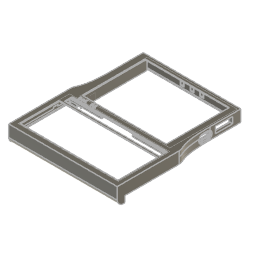
sol.01 (Autodesk Fusion 360 design; units mm, degrees)
Autodesk Fusion 360 part; units mm, degrees
note: some values were not read from the file. Set by a fixed rule: which face or edge a step refers to.
(part 1 of 2)
sketch "Sketch1" plane through (0, 0, 0) normal (0, 0, 1) x (1, 0, 0)
  line L0 (11.705, 132.02) -> (105.005, 132.02)
  line L1 (105.005, 132.02) -> (105.005, 61.35)
  line L2 (105.005, 61.35) -> (11.705, 61.35)
  line L3 (11.705, 61.35) -> (11.705, 132.02)
  line L4 (4.4, 58.89) -> (108.3, 58.89)
  line L5 (108.3, 58.89) -> (108.3, 5.46)
  line L6 (108.3, 5.46) -> (4.4, 5.46)
  line L7 (4.4, 5.46) -> (4.4, 58.89)
  line L8 (2, 62.35) -> (110.7, 62.35)
  line L9 (110.7, 62.35) -> (110.7, 2)
  line L10 (110.7, 2) -> (2, 2)
  line L11 (2, 2) -> (2, 62.35)
  line L12 (12.895, 129.09) -> (99.805, 129.09)
  line L13 (99.805, 129.09) -> (99.805, 63.79)
  line L14 (99.805, 63.79) -> (12.895, 63.79)
  line L15 (12.895, 63.79) -> (12.895, 129.09)
  line L16 (12.895, 129.09) -> (99.805, 63.79) construction
  line L17 (4.4, 58.89) -> (108.3, 5.46) construction
  line L18 (2, 62.35) -> (110.7, 2) construction
  line L19 (56.35, 96.44) -> (56.35, 32.175) construction
  line L20 (0, 0) -> (112.7, 0)
  line L21 (5.695, 64.35) -> (107.005, 64.35) construction
  line L22 (107.005, 134.02) -> (107.005, 70.045)
  line L23 (5.695, 134.02) -> (5.695, 70.045)
  line L24 (112.7, 0) -> (112.7, 64.35)
  line L25 (0, 64.35) -> (0, 0)
  line L26 (107.005, 134.02) -> (5.695, 134.02)
  line L27 (0, 64.35) -> (5.695, 70.045)
  line L28 (5.695, 64.35) -> (7.3315, 64.35) construction
  line L29 (112.7, 64.35) -> (107.005, 70.045)
  line L30 (107.005, 64.35) -> (105.9795, 64.35) construction
  line L31 (112.7, 64.35) -> (107.005, 64.35) construction
  line L32 (107.005, 64.35) -> (112.7, 64.35) construction
  line L33 (0, 64.35) -> (5.695, 64.35) construction
  line L34 (5.695, 70.045) -> (5.695, 64.35) construction
  line L35 (107.005, 70.045) -> (107.005, 64.35) construction
  line L36 (0, 64.35) -> (5.695, 64.35) construction
  line L37 (107.25, 47.24) -> (5.45, 47.24)
  line L38 (5.45, 47.24) -> (5.45, 6.29)
  line L39 (5.45, 6.29) -> (107.25, 6.29)
  line L40 (107.25, 6.29) -> (107.25, 47.24)
  line L41 (107.25, 57.36) -> (8.65, 57.36)
  line L42 (8.65, 57.36) -> (8.65, 49.36)
  line L43 (8.65, 49.36) -> (107.25, 49.36)
  line L44 (107.25, 49.36) -> (107.25, 57.36)
  line L45 (0, 64.35) -> (0, 70.045) construction
  line L46 (0, 70.045) -> (5.695, 70.045) construction
  line L47 (5.695, 70.045) -> (5.695, 102.0325) construction
  spline S0 degree 3 poles (0, 64.35) (0, 70.045) (5.695, 70.045) (5.695, 102.0325) knots 0 0 0 0 1 1 1 1
  line L48 (112.7, 64.35) -> (112.7, 70.045) construction
  line L49 (112.7, 70.045) -> (107.005, 70.045) construction
  line L50 (107.005, 70.045) -> (107.005, 102.0325) construction
  spline S1 degree 3 poles (112.7, 64.35) (112.7, 70.045) (107.005, 70.045) (107.005, 102.0325) knots 0 0 0 0 1 1 1 1
  point P0 (56.35, 96.44)
  point P1 (56.35, 32.175)
  point P2 (56.35, 32.175)
  dimension "d1" = 93.3
  dimension "d2" = 70.67
  dimension "d3" = 103.9
  dimension "d4" = 53.43
  dimension "d5" = 108.7
  dimension "d6" = 60.35
  dimension "d7" = 86.91
  dimension "d8" = 65.3
  dimension "d9" = 67.74
  dimension "d10" = 88.1
  dimension "d11" = 1
  dimension "d12" = 2
  dimension "d14" = 2
  dimension "d17" = 2
  dimension "d19" = 45
  dimension "d20" = 45
  dimension "d21" = 2
  dimension "d22" = 2
  dimension "d45" = 40.95
  dimension "d46" = 101.8
  dimension "d47" = 0.83
  dimension "d48" = 1.05
  dimension "d49" = 8
  dimension "d50" = 98.6
  dimension "d52" = 1.53
  dimension "d54" = 1.05
  dimension "d55" = 2
  constraint horizontal L0
  constraint vertical L1
  constraint horizontal L2
  constraint vertical L3
  constraint horizontal L4
  constraint vertical L5
  constraint horizontal L6
  constraint vertical L7
  constraint horizontal L8
  constraint vertical L9
  constraint horizontal L10
  constraint vertical L11
  constraint horizontal L12
  constraint vertical L13
  constraint horizontal L14
  constraint vertical L15
  constraint midpoint L16 P0
  constraint midpoint L17 P2
  constraint midpoint L18 P2
  constraint coincident P0 L19.start
  constraint coincident P2 P1
  constraint coincident P2 L19
  constraint vertical L19
  constraint horizontal L20
  constraint vertical L24
  constraint perpendicular L21 L24
  constraint perpendicular L21 L22
  constraint perpendicular L21 L23
  constraint vertical L25
  constraint horizontal L28
  constraint horizontal L30
  constraint perpendicular L24 L32
  constraint perpendicular L21 L34
  constraint perpendicular L21 L35
  constraint perpendicular L24 L36
  constraint equal L31 L36
  constraint coincident L20.start L25.end
  constraint horizontal L37
  constraint vertical L38
  constraint horizontal L39
  constraint vertical L40
  constraint horizontal L41
  constraint vertical L42
  constraint horizontal L43
  constraint vertical L44
  constraint vertical L45
  constraint coincident L23.end L27.end
  constraint horizontal L46
  constraint midpoint L23 L47.end
  constraint vertical L48
  constraint coincident L22.end L29.end
  constraint horizontal L49
  constraint midpoint L22 L50.end
  measures "d1" distance of L0.start L0.end
  measures "d2" distance of L0.start L2.end
  measures "d3" distance of L4.start L4.end
  measures "d4" distance of L4.start L6.end
  measures "d5" distance of L8.start L8.end
  measures "d6" distance of L8.start L10.end
  measures "d7" distance of L12.start L12.end
  measures "d8" distance of L12.start L14.end
  measures "d9" distance of L2 L12
  measures "d10" distance of L3 L13
  measures "d11" distance of L2 L8
  measures "d12" distance of L9 L24
  measures "d14" distance of L10 L20
  measures "d17" distance of L8 L21
  measures "d19" angle of L27 L28
  measures "d20" angle of L29 L30
  measures "d21" distance of L11 L25
  measures "d22" distance of L0 L26
  measures "d45" distance of L37.start L39.end
  measures "d46" distance of L37.start L37.end
  measures "d47" distance of L6 L39
  measures "d48" distance of L5 L40
  measures "d49" distance of L41.end L42.end
  measures "d50" distance of L41.start L41.end
  measures "d52" distance of L4 L41
  measures "d54" distance of L5 L44
  measures "d55" distance of L1 L22
sketch "Sketch2" plane through (0, 0, 0) normal (1, 0, 0) x (0, 1, 0)
  line L0 (64.35, 0) -> (70.045, 0)
  line L1 (64.35, 0) -> (0, 0)
  line L2 (0, 0) -> (64.35, 0)
  line L3 (64.35, 0) -> (70.045, 0)
  line L4 (134.02, 0) -> (70.045, 0)
  line L5 (134.02, 0) -> (70.045, 0)
  line L6 (0, 0) -> (134.52, 0)
  line L7 (134.52, 0) -> (134.52, 12.2)
  line L8 (134.52, 12.2) -> (0, 12.2)
  line L9 (0, 12.2) -> (0, 0)
  line L10 (129.09, 0) -> (63.79, 0)
  line L11 (63.79, 0) -> (129.09, 0)
  line L12 (129.55, 12.2) -> (66.3267, 12.2)
  line L13 (129.55, 12.2) -> (64.25, 12.2)
  line L14 (64.25, 12.2) -> (64.25, 11.45)
  line L15 (64.25, 11.45) -> (129.55, 11.45)
  line L16 (129.55, 11.45) -> (129.55, 12.2)
  line L17 (132.02, 0) -> (62.35, 0)
  line L18 (62.35, 0) -> (62.35, 11.45)
  line L19 (62.35, 11.45) -> (132.02, 11.45)
  line L20 (132.02, 11.45) -> (132.02, 0)
  line L21 (5.46, 0) -> (58.89, 0)
  line L22 (58.89, 0) -> (5.46, 0)
  line L23 (58.89, 0) -> (62.35, 0)
  line L24 (62.35, 0) -> (62.35, 6.9)
  line L25 (62.35, 6.9) -> (58.89, 6.9)
  line L26 (58.89, 6.9) -> (58.89, 0)
  line L27 (62.35, 0) -> (2, 0)
  line L28 (2, 0) -> (62.35, 0)
  line L29 (2, 0) -> (6.61, 0)
  line L30 (6.61, 0) -> (6.61, 6.9)
  line L31 (6.61, 6.9) -> (2, 6.9)
  line L32 (2, 6.9) -> (2, 0)
  line L33 (58.89, 0) -> (6.61, 0)
  line L34 (6.61, 0) -> (6.61, 12.2)
  line L35 (6.61, 12.2) -> (58.89, 12.2)
  line L36 (58.89, 12.2) -> (58.89, 0)
  point P0 (134.02, 0)
  point P1 (61.35, 0)
  point P2 (132.02, 0)
  point P3 (63.79, 0)
  point P4 (129.09, 0)
  point P5 (5.46, 0)
  point P6 (58.89, 0)
  point P7 (62.35, 0)
  point P8 (2, 0)
  dimension "d27" = 0.75
  dimension "d28" = 5.3
  dimension "d29" = 5.3
  dimension "d213" = 12.2
  constraint horizontal L6
  constraint vertical L7
  constraint horizontal L8
  constraint vertical L9
  constraint coincident L1.end L2.start
  constraint coincident L8 L12.start
  constraint coincident L8 L12.end
  constraint horizontal L13
  constraint vertical L14
  constraint horizontal L15
  constraint vertical L16
  constraint horizontal L17
  constraint vertical L18
  constraint horizontal L19
  constraint vertical L20
  constraint coincident P2 L17.start
  constraint coincident L14.end L19
  constraint horizontal L23
  constraint vertical L24
  constraint horizontal L25
  constraint vertical L26
  constraint coincident L18 L24.end
  constraint coincident P6 L21.end
  constraint horizontal L29
  constraint vertical L30
  constraint horizontal L31
  constraint vertical L32
  constraint coincident P8 L27.end
  constraint horizontal L33
  constraint vertical L34
  constraint horizontal L35
  constraint vertical L36
  constraint coincident L8 L34.end
  measures "d27" distance of L12.start L15.end
  measures "d28" distance of L8 L25
  measures "d29" distance of L8 L31
  measures "d213" distance of L1.end L8.end
extrude "Extrude1" add sketch "Sketch1" along normal up to surface (6.9 mm away) contours L20 L22 L23 L24 L25 L26 L27 L29 | L23 L27 S0 | L22 L29 S1 makes body 1
extrude "Extrude2" add sketch "Sketch1" along normal up to surface (4.55 mm away) from surface at 6.9 contours L1 L2 L3 L8 | L1 L2 L3 L8 L9 L10 L11 | L20 L22 L23 L24 L25 L26 L27 L29 | L23 L27 S0 | L22 L29 S1 bodies 1
extrude "Extrude3" add sketch "Sketch1" along normal up to surface (0.75 mm away) from surface at 11.45 contours L0 L1 L3 L8 | L1 L2 L3 L8 | L1 L2 L3 L8 L9 L10 L11 | L4 L5 L6 L7 | L20 L22 L23 L24 L25 L26 L27 L29 | L23 L27 S0 | L22 L29 S1 bodies 1
chamfer "Chamfer1" distance 15.9974 distance2 5.557 1 edges at (105.005, 62.35, 3.45) measured on face at (105.005, 108.7967, 6.1167) tangent chain off on bodies 1
sketch "Sketch4" plane through (0, 0, 6.9) normal (0, 0, -1) x (1, 0, 0)
  line L0 (2, -62.35) -> (11.705, -62.35)
  line L1 (11.705, -62.35) -> (105.005, -62.35)
  line L2 (105.005, -62.35) -> (105.005, -78.3474)
  line L3 (105.005, -78.3474) -> (110.562, -62.35)
  line L4 (110.562, -62.35) -> (110.7, -62.35)
  line L5 (110.7, -62.35) -> (110.7, -2)
  line L6 (110.7, -2) -> (2, -2)
  line L7 (2, -2) -> (2, -62.35)
  line L8 (108.3, -5.46) -> (108.3, -58.89)
  line L9 (108.3, -58.89) -> (4.4, -58.89)
  line L10 (4.4, -58.89) -> (4.4, -5.46)
  line L11 (4.4, -5.46) -> (108.3, -5.46)
  line L12 (108.3, -45.623) -> (114.9584, -45.623) construction
  line L13 (108.3, -43.4637) -> (114.9584, -43.4637) construction
  line L14 (4.4, -5.46) -> (108.3, -5.46)
  line L15 (4.4211, -57.9322) -> (38.5072, -57.9322)
  line L16 (4.4211, -5.46) -> (4.4211, -18.9792)
  line L17 (18.0884, -18.9792) -> (4.4211, -18.9792)
  line L18 (18.0884, -18.9792) -> (18.0884, -23.4975)
  line L19 (18.0884, -23.4975) -> (46.0418, -23.4975)
  line L20 (46.0418, -23.4975) -> (46.0418, -35.9296)
  line L21 (46.0418, -35.9296) -> (55.7614, -35.9296)
  line L22 (55.7614, -35.9296) -> (55.7614, -27.3401)
  line L23 (55.7614, -27.3401) -> (96.5989, -27.3401)
  line L24 (96.5989, -27.3401) -> (96.5989, -37.5118)
  line L25 (96.5989, -37.5118) -> (70.3785, -37.5118)
  line L26 (70.3785, -37.5118) -> (70.3785, -62.35)
  line L27 (38.5072, -62.35) -> (70.3785, -62.35)
  line L28 (70.3785, -62.35) -> (70.3785, -56.725)
  line L29 (38.5072, -56.725) -> (38.5072, -62.35)
  line L30 (70.3785, -56.725) -> (38.5072, -56.725)
  line L31 (4.0998, -44.4778) -> (-1.4115, -38.9664)
  line L32 (4.0998, -44.4778) -> (4.0998, -44.999)
  line L33 (-1.4116, -50.5103) -> (-1.4115, -38.9664)
  line L34 (4.0998, -44.999) -> (-1.4116, -50.5103)
  line L35 (2, -47.0988) -> (4.4, -47.0988)
  line L36 (2, -42.378) -> (4.4, -42.3611)
  line L37 (4.4211, -18.9792) -> (4.4211, -57.9322)
  line L38 (4.4, -47.0988) -> (4.4211, -47.0988)
  line L39 (4.4, -42.3611) -> (4.4211, -42.3611)
  line L40 (70.3785, -57.9438) -> (108.3, -57.9438)
  line L41 (108.3, -5.46) -> (108.3, -57.9438)
  line L42 (108.2, -57.9438) -> (108.2, -5.46)
  line L43 (108.3, -5.56) -> (4.4211, -5.56)
  dimension "d90" = 0.1
  dimension "d91" = 0.1
  constraint horizontal L12
  constraint coincident L8 L12.start
  constraint horizontal L13
  constraint coincident L8 L13.start
  constraint coincident L10.end L11.start
  constraint coincident L8.start L11.end
  constraint coincident L15.end L29
  constraint perpendicular L15 L29
  constraint parallel L26 L28
  constraint coincident L34 L35.start
  constraint coincident L7 L35.start
  constraint coincident L10 L35.end
  constraint coincident L31 L36.start
  constraint coincident L7 L36.start
  constraint coincident L10 L36.end
  constraint coincident L14 L16.start
  constraint vertical L16
  constraint horizontal L17
  constraint vertical L18
  constraint horizontal L19
  constraint vertical L20
  constraint horizontal L21
  constraint vertical L22
  constraint horizontal L23
  constraint vertical L24
  constraint horizontal L25
  constraint vertical L26
  constraint horizontal L30
  constraint vertical L29
  constraint vertical L37
  constraint coincident L37 L38.end
  constraint perpendicular L37 L38
  constraint coincident L37 L39.end
  constraint perpendicular L37 L39
  constraint coincident L26 L40.start
  constraint coincident L8 L40.end
  constraint perpendicular L8 L40
  constraint coincident L40 L42.start
  constraint coincident L14 L42.end
  constraint perpendicular L14 L42
  constraint coincident L41 L43.start
  constraint coincident L16 L43.end
  constraint perpendicular L16 L43
  measures "d90" distance of L14 L43
  measures "d91" distance of L41 L42
box "BoxPrimitive6" add length 1.8 width 103.9 height 1 placed x (0, 0, 1) y (-1, 0, 0) z (0, -1, 0) at (108.3, 58.89, 6.9) bodies 1
extrude "Extrude4" cut sketch "Sketch4" against normal blind 1.8 contours L1 L9 L26 L27 L28 L29 | L9 L26 L28 L29 L30 bodies 1
extrude "Extrude5" cut sketch "Sketch4" along normal blind 0.9639 and the other way blind 1.628 contours L7 L31 L33 L34 | L7 L31 L32 L34 | L10 L31 L32 L34 L35 L36 bodies 1
extrude "Extrude6" add sketch "Sketch4" against normal blind 1 separate body contours L16 L17 L18 L19 L20 L21 L22 L23 L24 L25 L26 L28 L40 L42 L43 makes body 2
sketch "Sketch6" plane through (0, 0, 11.45) normal (0, 0, -1) x (1, 0, 0)
  line L0 (99.805, -63.79) -> (99.805, -129.09)
  line L1 (99.805, -129.09) -> (12.895, -129.09)
  line L2 (12.895, -129.09) -> (12.895, -63.79)
  line L3 (12.895, -63.79) -> (99.805, -63.79)
  line L4 (105.005, -62.35) -> (11.705, -62.35)
  line L5 (11.705, -62.35) -> (11.705, -132.02)
  line L6 (11.705, -132.02) -> (105.005, -132.02)
  line L7 (105.005, -132.02) -> (105.005, -62.35)
  line L8 (105.005, -102.5509) -> (110.748, -108.2939)
  line L9 (105.005, -102.5509) -> (113.1461, -102.5509) construction
  line L10 (105.005, -91.9597) -> (113.3226, -83.6421)
  line L11 (105.005, -102.5509) -> (105.005, -91.9597)
  line L12 (110.748, -108.2939) -> (110.748, -86.2167)
  line L13 (105.005, -123.4211) -> (110.0091, -128.4252)
  line L14 (105.005, -123.4211) -> (112.0734, -123.4211) construction
  line L15 (105.005, -123.4211) -> (105.005, -109.5726)
  line L16 (70.1416, -132.02) -> (66.6021, -132.02)
  line L17 (66.6021, -132.02) -> (66.6021, -134.703)
  line L18 (66.6021, -134.703) -> (70.1416, -134.703)
  line L19 (70.1416, -134.703) -> (70.1416, -132.02)
  line L20 (60.0287, -132.02) -> (56.5904, -132.02)
  line L21 (56.5904, -132.02) -> (56.5904, -135.0064)
  line L22 (56.5904, -135.0064) -> (60.0287, -135.0064)
  line L23 (60.0287, -135.0064) -> (60.0287, -132.02)
  line L24 (49.8148, -132.02) -> (46.2753, -132.02)
  line L25 (46.2753, -132.02) -> (46.2753, -134.6019)
  line L26 (46.2753, -134.6019) -> (49.8148, -134.6019)
  line L27 (49.8148, -134.6019) -> (49.8148, -132.02)
  line L28 (11.705, -62.35) -> (10.905, -62.35)
  line L29 (10.905, -62.35) -> (10.905, -78.35)
  line L30 (10.905, -78.35) -> (6.705, -78.35)
  line L31 (6.705, -78.35) -> (6.705, -72.35)
  line L32 (6.705, -72.35) -> (8.405, -72.35)
  line L33 (8.405, -72.35) -> (8.405, -62.35)
  line L34 (8.405, -62.35) -> (11.705, -62.35)
  line L35 (8.405, -62.35) -> (10.905, -62.35)
  line L36 (6.705, -75.35) -> (5.2663, -75.35)
  line L37 (11.705, -63.3036) -> (10.905, -63.3036)
  line L38 (105.005, -109.5726) -> (107.7995, -106.7781)
  line L39 (107.7995, -106.7781) -> (107.7995, -126.2156)
  dimension "d73" = 45
  dimension "d74" = 90
  dimension "d75" = 45
  dimension "d76" = 0.8
  dimension "d77" = 4.2
  dimension "d78" = 6
  dimension "d79" = 16
  dimension "d80" = 2.5
  constraint horizontal L9
  constraint coincident L7 L8.start
  constraint coincident L7 L10.start
  constraint coincident L10 L12.end
  constraint perpendicular L9 L12
  constraint horizontal L14
  constraint coincident L7 L13.start
  constraint coincident L7 L15.end
  constraint horizontal L16
  constraint vertical L17
  constraint horizontal L18
  constraint vertical L19
  constraint coincident L6 L16.start
  constraint horizontal L20
  constraint vertical L21
  constraint horizontal L22
  constraint vertical L23
  constraint coincident L6 L20.start
  constraint horizontal L24
  constraint vertical L25
  constraint horizontal L26
  constraint vertical L27
  constraint coincident L6 L24.start
  constraint coincident L4.end L5.start
  constraint perpendicular L5 L28
  constraint perpendicular L28 L29
  constraint perpendicular L29 L30
  constraint perpendicular L30 L31
  constraint perpendicular L31 L32
  constraint perpendicular L28 L33
  constraint perpendicular L5 L34
  constraint midpoint L31 L36.start
  constraint perpendicular L31 L36
  constraint coincident L5 L37.start
  constraint coincident L29 L37.end
  constraint perpendicular L29 L37
  constraint perpendicular L8 L38
  constraint coincident L13 L39.end
  constraint vertical L39
  measures "d73" angle of L8 L9
  measures "d74" angle of L8 L10
  measures "d75" angle of L13 L14
  measures "d76" distance of L4.end L28.end
  measures "d77" distance of L29.end L30.end
  measures "d78" distance of L30.end L31.end
  measures "d79" distance of L30 L35
  measures "d80" distance of L29 L33
extrude "Extrude7" cut sketch "Sketch6" along normal blind 16.15 from surface at 4.55 contours L5 L28 L29 L34 L37 | L29 L30 L31 L32 L33 L34 L35 bodies 1
sketch "Sketch7" plane through (6.705, 0, 0) normal (1, 0, 0) x (0, 1, 0)
  line L0 (78.35, 6.9) -> (72.35, 6.9)
  line L1 (72.35, 6.9) -> (72.35, 0)
  line L2 (78.35, 0) -> (78.35, 6.9)
  circle A0 centre (75.35, 3.0769) radius 2
  line L3 (77.35, 3.0769) -> (77.35, -1.1276)
  line L4 (73.35, 3.0769) -> (73.35, -1.1276)
  line L5 (73.35, -1.1276) -> (77.35, -1.1276)
  line L6 (72.35, 0) -> (78.35, 0)
  dimension "d84" = 4
  constraint coincident A0 L3.start
  constraint tangent A0 L3
  constraint coincident A0 L4.start
  constraint tangent A0 L4
  constraint perpendicular L3 L5
  measures "d84" diameter of A0
extrude "Extrude8" cut sketch "Sketch7" against normal blind 8.5544 contours A0 L3 L4 L6 | L3 L4 L5 L6 | A0 bodies 1
extrude "Extrude9" cut sketch "Sketch6" along normal blind 4 from surface at 3.2 contours L7 L13 L15 L38 L39 | L6 L24 L25 L26 L27 | L6 L20 L21 L22 L23 | L6 L16 L17 L18 L19 bodies 1
sketch "Sketch8" plane through (107.005, 0, 0) normal (1, 0, 0) x (0, 1, 0)
  line L0 (125.4211, 8.25) -> (125.4211, 4.25)
  line L1 (125.4211, 4.25) -> (107.5726, 4.25)
  line L2 (107.5726, 4.25) -> (107.5726, 8.25)
  line L3 (107.5726, 8.25) -> (125.4211, 8.25)
  line L4 (102.0325, 0) -> (134.02, 0)
  line L5 (134.02, 0) -> (134.02, 12.2)
  line L6 (134.02, 12.2) -> (102.0325, 12.2)
  line L7 (99.6683, 8.953) -> (94.3183, 8.953)
  arc A0 (94.3183, 8.953) -> (94.3183, 1.603) centre (94.3183, 5.278) ccw
  line L8 (94.3183, 1.603) -> (99.6683, 1.603)
  arc A1 (99.6683, 1.603) -> (99.6683, 8.953) centre (99.6683, 5.278) ccw
  line L9 (103.3433, 5.278) -> (90.6433, 5.278) construction
  line L10 (101.5433, 6.943) -> (92.4433, 6.943)
  line L11 (92.4433, 6.943) -> (92.4433, 3.613)
  line L12 (92.4433, 3.613) -> (101.5433, 3.613)
  line L13 (101.5433, 3.613) -> (101.5433, 6.943)
  line L14 (101.5433, 6.943) -> (92.4433, 3.613) construction
  line L15 (92.4433, 6.943) -> (101.5433, 3.613) construction
  line L16 (92.4433, 6.943) -> (91.0421, 6.943)
  line L17 (101.5433, 6.943) -> (102.9445, 6.943)
  line L18 (99.6683, 9.6498) -> (94.3183, 9.6498)
  arc A2 (94.3183, 9.6498) -> (94.3183, 0.9062) centre (94.3183, 5.278) ccw
  line L19 (94.3183, 0.9062) -> (99.6683, 0.9062)
  arc A3 (99.6683, 0.9062) -> (99.6683, 9.6498) centre (99.6683, 5.278) ccw
  line L20 (99.6683, 5.278) -> (94.3183, 5.278) construction
  line L21 (102.9445, 6.943) -> (103.7106, 6.943)
  line L22 (91.0421, 6.943) -> (90.276, 6.943)
  line L23 (91.9433, 7.443) -> (102.0433, 7.443)
  line L24 (102.0433, 7.443) -> (102.0433, 3.113)
  line L25 (102.0433, 3.113) -> (91.9433, 3.113)
  line L26 (91.9433, 3.113) -> (91.9433, 7.443)
  line L27 (91.9433, 7.443) -> (102.0433, 3.113) construction
  line L28 (102.0433, 7.443) -> (91.9433, 3.113) construction
  line L29 (102.0325, 12.2) -> (102.0325, 6.9)
  line L30 (102.0325, 6.9) -> (102.0325, 0)
  point P0 (96.9933, 5.278)
  point P1 (96.9933, 5.278)
  dimension "d92" = 7.35
  dimension "d93" = 9.1
  dimension "d94" = 3.33
  dimension "d97" = 10.1
  dimension "d98" = 4.33
  constraint tangent L7 A0
  constraint tangent A0 L8
  constraint parallel L7 L8
  constraint tangent L8 A1
  constraint tangent L7 A1
  constraint coincident A1 L9.start
  constraint coincident A0 L9.end
  constraint coincident A0.centre L9
  constraint coincident A1.centre L9
  constraint horizontal L9
  constraint horizontal L10
  constraint perpendicular L10 L11
  constraint parallel L10 L12
  constraint parallel L11 L13
  constraint coincident L14 P1
  constraint coincident L15 P1
  constraint midpoint L9 P1
  constraint coincident A0 L16.end
  constraint perpendicular L11 L16
  constraint coincident A1 L17.end
  constraint perpendicular L13 L17
  constraint tangent L18 A2
  constraint tangent A2 L19
  constraint parallel L18 L19
  constraint tangent L19 A3
  constraint tangent L18 A3
  constraint coincident A0.centre A2.centre
  constraint parallel L9 L20
  constraint coincident A1.centre A3.centre
  constraint coincident A3 L21.end
  constraint parallel L17 L21
  constraint coincident A2 L22.end
  constraint parallel L16 L22
  constraint horizontal L23
  constraint perpendicular L23 L24
  constraint parallel L23 L25
  constraint parallel L24 L26
  constraint coincident L27 P1
  constraint coincident L28 P1
  constraint coincident P1 P0
  measures "d92" diameter of A0
  measures "d93" distance of L11.end L12.end
  measures "d94" distance of L10.end L11.end
  measures "d97" distance of L24.end L25.end
  measures "d98" distance of L23.end L24.end
extrude "Extrude10" cut sketch "Sketch8" along normal blind -1.64 and the other way blind -1.013 contours A1 L17 L24 L25 L30 | A0 L8 A1 L16 L25 L26 L30 | A1 L17 L23 L24 L29 | L17 L24 L25 L29 L30 | L11 L12 L13 L16 L17 L25 L26 L29 L30 | L7 A0 A1 L16 L23 L26 L29 | L17 L23 L24 L29 | L10 L16 L17 L23 L26 L29 | L10 L11 L12 L13 bodies 1
extrude "Extrude11" add sketch "Sketch8" against normal blind 1.5 from surface at -1.64 contours L17 L24 L25 L29 L30 | L11 L12 L13 L16 L17 L25 L26 L29 L30 bodies 1
extrude "Extrude12" cut sketch "Sketch8" along normal blind -4.864 and the other way blind -7.446 contours L10 L11 L12 L13 bodies 1
sketch "Sketch9" plane through (70.1416, 0, 0) normal (-1, 0, 0) x (0, -1, 0)
  line L0 (-134.02, 8.25) -> (-134.02, 4.25)
  line L1 (-134.02, 4.25) -> (-132.02, 4.25)
  line L2 (-132.02, 4.25) -> (-132.02, 8.25)
  line L3 (-132.02, 8.25) -> (-134.02, 8.25)
  line L4 (-132.02, 4.25) -> (-132.02, 7.6162)
  line L5 (-134.8367, 7.6162) -> (-134.8367, 4.9116)
  line L6 (-134.8367, 4.9116) -> (-132.4955, 4.9116)
  line L7 (-132.02, 4.25) -> (-132.02, 7.6162)
  line L8 (-132.02, 7.6162) -> (-132.02, 8.25)
  line L9 (-132.02, 7.6162) -> (-132.3677, 7.6162) construction
  line L10 (-132.3677, 7.6162) -> (-132.3677, 7.9331) construction
  line L11 (-132.3677, 8.25) -> (-132.02, 8.25)
  line L12 (-132.02, 8.25) -> (-132.02, 7.6162)
  line L13 (-132.3677, 8.25) -> (-132.6161, 8.25)
  line L14 (-132.6161, 8.25) -> (-132.6161, 7.6162) construction
  line L15 (-132.6161, 7.6162) -> (-132.3677, 7.6162) construction
  line L16 (-132.3677, 7.6162) -> (-132.3677, 8.25) construction
  arc A0 (-132.6161, 7.6162) -> (-132.6161, 8.25) centre (-132.694, 7.9331) ccw
  line L17 (-132.3677, 7.9331) -> (-132.3677, 8.25) construction
  line L18 (-134.8367, 7.6162) -> (-134.02, 7.6162)
  line L19 (-132.6161, 7.6162) -> (-132.02, 7.6162) construction
  line L20 (-134.02, 7.6162) -> (-132.6161, 7.6162)
  line L21 (-132.4955, 4.9116) -> (-132.02, 4.9027)
  constraint coincident L1.end L2.start
  constraint coincident L2 L4.end
  constraint parallel L0 L5
  constraint perpendicular L0 L6
  constraint perpendicular L4 L18
  constraint coincident L2.end L3.start
  constraint horizontal L9
  constraint vertical L10
  constraint horizontal L11
  constraint vertical L12
  constraint coincident L3 L11.start
  constraint horizontal L13
  constraint vertical L14
  constraint horizontal L15
  constraint vertical L16
  constraint coincident L14.end L18
  constraint tangent L16 A0
  constraint coincident A0 L10.end
  constraint vertical L17
  constraint coincident L0 L18.end
  constraint coincident L4 L21.end
extrude "Extrude13" add sketch "Sketch9" along normal blind 2.75 from surface at 0.4 separate body contours L0 L2 L3 L4 L6 L7 L8 L11 L12 L13 A0 L20 L21 | L0 L5 L6 L18 makes body 3
copy_body "CopyPasteBodies1" bodies 3 makes body 4
move_body "Move1" bodies 4 to x (1, 0, 0) y (0, 1, 0) z (0, 0, 1) at (-10.0117, 0, 0)
copy_body "CopyPasteBodies2" bodies 3 makes body 5
move_body "Move2" bodies 5 to x (1, 0, 0) y (0, 1, 0) z (0, 0, 1) at (-20.3268, 0, 0)
combine "Combine1" operation add target body 1 tool bodies 5 4 3
move_face "OffsetFaces1" offset -0.196 6 faces at (70.1416, 133.3533, 6.9167) (60.0287, 133.3533, 6.9167) (49.8148, 133.3533, 6.9167) (66.6021, 132.6867, 6.9167) (56.5904, 132.6867, 6.9167) (46.2753, 132.6867, 6.9167) on bodies 1
move_face "OffsetFaces2" offset 0.243 3 faces at (68.8249, 134.8367, 6.7147) (58.8132, 134.8367, 6.7147) (48.4981, 134.8367, 6.7147) on bodies 1
chamfer "Chamfer2" distance 0.5883 angle 45 12 edges at (48.0398, 135.0797, 7.6162) (46.6648, 135.0797, 6.2639) (48.0398, 135.0797, 4.9116) (49.4148, 135.0797, 6.2639) (58.3549, 135.0797, 7.6162) (56.9799, 135.0797, 6.2639) (58.3549, 135.0797, 4.9116) (59.7299, 135.0797, 6.2639) (68.3666, 135.0797, 7.6162) (66.9916, 135.0797, 6.2639) (68.3666, 135.0797, 4.9116) (69.7416, 135.0797, 6.2639) tangent chain off on bodies 1
move_face "MoveFace2" by (0, 0, 0.2611) 1 faces at (106.3383, 114.1887, 4.25) on bodies 1
sketch "Sketch17" plane through (112.7, 0, 0) normal (1, 0, 0) x (0, 1, 0)
  line L0 (0, 12.2) -> (0, 0)
  line L1 (0, 0) -> (64.35, 0)
  line L2 (64.35, 0) -> (64.35, 6.9)
  line L3 (64.35, 6.9) -> (64.35, 12.2)
  line L4 (64.35, 12.2) -> (0, 12.2)
  line L5 (8.1693, -5.2409) -> (56.1807, -5.2409)
  arc A0 (56.1807, -5.2409) -> (56.1807, 6.8891) centre (56.1807, 0.8241) ccw
  line L6 (56.1807, 6.8891) -> (8.1693, 6.8891)
  arc A1 (8.1693, 6.8891) -> (8.1693, -5.2409) centre (8.1693, 0.8241) ccw
  line L7 (2.1043, 0.8241) -> (62.2457, 0.8241) construction
  line L8 (2, 0) -> (62.8584, 0) construction
  line L9 (62.8584, 0) -> (62.8584, -5.4) construction
  line L10 (62.8584, -5.4) -> (2, -5.4) construction
  line L11 (2, -5.4) -> (2, 0) construction
  arc A2 (2, 0) -> (8.1693, -5.4) centre (8.1693, 0.8241) ccw
  arc A3 (0, 0) -> (6.4, -6.4) centre (6.4, 0) ccw
  line L12 (6.4, -6.4) -> (56.1396, -6.4)
  line L13 (8.1693, -5.4) -> (56.1807, -5.4)
  arc A4 (56.1807, -5.4) -> (62.35, 0) centre (56.1807, 0.8241) ccw
  line L14 (56.1807, 0.8241) -> (56.1807, -5.4) construction
  line L15 (8.1693, 0.8241) -> (8.1693, -5.4) construction
  line L16 (8.1693, -5.4) -> (8.1693, -6.4) construction
  line L17 (8.1693, -5.9) -> (6.5592, -5.9)
  line L18 (6.5592, -5.9) -> (6.5592, -5.1881)
  line L19 (8.1693, -5.4) -> (6.5592, -5.4)
  line L20 (8.1693, -5.9) -> (8.1693, -6.4)
  line L21 (62.35, 0) -> (134.02, 0)
  line L22 (134.02, 0) -> (134.02, -1.3)
  line L23 (56.1396, -6.4) -> (64.35, -6.4) construction
  line L24 (64.35, -6.4) -> (64.35, 0) construction
  line L25 (134.02, -1.3) -> (64.35, -1.3) construction
  line L26 (56.1396, -6.4) -> (64.35, -6.4) construction
  line L27 (64.35, -6.4) -> (64.35, -1.3) construction
  line L28 (64.35, -1.3) -> (99.185, -1.3) construction
  spline S0 degree 3 poles (56.1396, -6.4) (64.35, -6.4) (64.35, -1.3) (99.185, -1.3) knots 0 0 0 0 1 1 1 1
  line L29 (99.185, -1.3) -> (134.02, -1.3)
  spline S1 degree 3 poles (56.1807, -5.4) (64.391, -5.4) (64.391, -0.293) (98.185, 0) knots 0 0 0 0 1 1 1 1
  line L30 (56.1807, -5.4) -> (64.391, -5.4) construction
  line L31 (64.391, -5.4) -> (64.391, -0.293) construction
  line L32 (64.391, -0.293) -> (98.185, 0) construction
  line L33 (8.1693, -5.9) -> (8.1693, 0)
  line L34 (2, 0) -> (8.1693, 0)
  point P0 (2, 0)
  point P1 (62.35, 0)
  point P2 (134.02, 0)
  dimension "d214" = 12.13
  dimension "d220" = 5.4
  dimension "d222" = 1.3
  dimension "d223" = 1
  constraint tangent L5 A0
  constraint tangent A0 L6
  constraint parallel L5 L6
  constraint tangent L6 A1
  constraint tangent L5 A1
  constraint coincident A1 L7.start
  constraint coincident A0 L7.end
  constraint coincident A0.centre L7
  constraint coincident A1.centre L7
  constraint horizontal L7
  constraint horizontal L8
  constraint vertical L9
  constraint horizontal L10
  constraint vertical L11
  constraint coincident P0 L8.start
  constraint coincident A1.centre A2.centre
  constraint coincident L0.end L1.start
  constraint coincident L8 A3.centre
  constraint tangent A3 L12
  constraint parallel L10 L12
  constraint tangent A2 L13
  constraint parallel L10 L13
  constraint coincident P1 A4.end
  constraint coincident A0.centre A4.centre
  constraint coincident L13.end A4
  constraint coincident L13.end A4.start
  constraint vertical L14
  constraint collinear L10 L13
  constraint coincident L12 L16.end
  constraint perpendicular L12 L16
  constraint midpoint L16 L17.start
  constraint perpendicular L16 L17
  constraint coincident A2 L18.end
  constraint perpendicular L10 L18
  constraint coincident L10 L19.end
  constraint coincident L18 L19.end
  constraint coincident P2 L21.end
  constraint perpendicular L21 L22
  constraint perpendicular L9 L23
  constraint coincident L1.end L2.start
  constraint perpendicular L21 L24
  constraint coincident L24 L25.end
  constraint perpendicular L24 L25
  constraint coincident L23.end L24.start
  constraint coincident L25.end L27.end
  constraint midpoint L25 L28.end
  constraint coincident L21 S1.end
  constraint coincident L10 L13.end
  constraint midpoint L21 S1.end
  constraint coincident L8 L33.end
  constraint coincident L15 L33.end
  measures "d214" diameter of A0
  measures "d220" distance of P0 L10.end
  measures "d222" distance of P2 L22.end
  measures "d223" distance of L12 L13
extrude "Extrude14" add sketch "Sketch17" against normal up to surface (108.7 mm away) from surface at -2 contours L1 A2 A3 L12 L17 L18 L20 bodies 1
extrude "Extrude15" add sketch "Sketch17" against normal up to surface (2 mm away) contours L1 A2 A3 L12 L17 L18 L20 | L1 A1 A2 L33 L34 | L1 A1 L33 L34 | A2 L18 L19 | L17 L18 L19 L33 bodies 1
extrude "Extrude16" add sketch "Sketch17" against normal up to surface (2 mm away) from surface at -110.7 contours L1 A2 A3 L12 L17 L18 L20 | L1 A1 A2 L33 L34 | L1 A1 L33 L34 | A2 L18 L19 | L17 L18 L19 L33 bodies 1
move_face "MoveFace3" by (0, 0, -0.1013) 3 faces at (48.7003, 132.6867, 4.25) (58.9479, 133.3533, 4.25) (69.0271, 133.3533, 4.25) on bodies 1
extrude "Extrude17" add sketch "Sketch17" along normal up to surface (112.7 mm away) from surface at -112.7 separate body contours L12 L13 L20 L21 L22 S0 L29 S1 L33 | L17 L18 L19 L33 makes body 6
sketch "Sketch20" plane through (0, 0, 0) normal (0, 0, 1) x (-1, 0, 0)
  line L0 (-112.7, -134.02) -> (0, -134.02)
  line L1 (0, -98.185) -> (-112.7, -98.185)
  line L2 (-107.005, -134.02) -> (-5.695, -134.02)
  line L3 (-11.705, -61.35) -> (-11.705, -132.02)
  line L4 (-11.705, -132.02) -> (-105.005, -132.02)
  line L5 (-105.005, -132.02) -> (-105.005, -61.35)
  line L6 (-107.005, -134.02) -> (-107.005, -70.045)
  line L7 (-105.005, -61.35) -> (-11.705, -61.35)
  spline S0 degree 3 poles (-112.7, -64.35) (-112.7, -70.045) (-107.005, -70.045) (-107.005, -102.0325) knots 0 0 0 0 1 1 1 1
  spline S1 degree 3 poles (0, -64.35) (0, -70.045) (-5.695, -70.045) (-5.695, -102.0325) knots 0 0 0 0 1 1 1 1
  line L8 (-5.695, -134.02) -> (-5.695, -70.045)
  line L9 (0, -134.02) -> (0, -98.185)
  line L10 (-112.7, -98.185) -> (-112.7, -134.02)
  spline S2 degree 3 poles (-2, -64.35) (-2, -65.2963) (-2.1743, -65.9372) (-2.553, -66.9153) (-3.145, -68.4443) (-4.2661, -70.649) (-5.2629, -74.5545) (-6.5675, -79.6654) (-7.695, -87.7291) (-7.695, -102.0325) knots 0 0 0 0 0.216963 0.216963 0.216963 0.556139 0.556139 0.556139 1 1 1 1
  spline S3 degree 3 poles (-110.7, -64.35) (-110.7, -65.2963) (-110.5257, -65.9372) (-110.147, -66.9153) (-109.555, -68.4443) (-108.4339, -70.649) (-107.4371, -74.5545) (-106.1325, -79.6654) (-105.005, -87.7291) (-105.005, -102.0325) knots 0 0 0 0 0.216963 0.216963 0.216963 0.556139 0.556139 0.556139 1 1 1 1
  line L11 (-5.695, -102.0325) -> (-5.695, -134.02)
  line L12 (-107.005, -134.02) -> (-5.695, -134.02)
  line L13 (-7.695, -132.02) -> (-7.695, -102.0325)
  line L14 (-7.695, -132.02) -> (-105.005, -132.02)
  line L15 (-105.005, -102.0325) -> (-105.005, -132.02)
  line L16 (0, -98.185) -> (0, -56.1807)
  line L17 (0, -56.1807) -> (0, -6.5592)
  line L18 (0, -6.5592) -> (-112.7, -6.5592)
  line L19 (-112.7, -6.5592) -> (-112.7, -56.1807)
  line L20 (-112.7, -56.1807) -> (-112.7, -98.185)
  line L21 (-2, -64.35) -> (-2, -6.5592)
  line L22 (-110.7, -64.35) -> (-110.7, -6.5592)
  line L23 (-107.005, -102.0325) -> (-107.005, -134.02)
  line L24 (-5.695, -102.0325) -> (-5.695, -134.02)
  line L25 (0, -8.1693) -> (-112.7, -8.1693)
  spline S4 degree 3 poles (-1, -64.35) (-1, -65.5895) (-1.2863, -66.469) (-1.7932, -67.7094) (-2.5642, -69.5962) (-3.8217, -72.1868) (-4.8446, -77.2142) (-5.8772, -82.2895) (-6.695, -89.879) (-6.695, -102.0325) knots 0 0 0 0 0.246494 0.246494 0.246494 0.621459 0.621459 0.621459 1 1 1 1
  line L26 (-6.695, -102.0325) -> (-6.695, -133.02)
  line L27 (-106.005, -133.02) -> (-6.695, -133.02)
  line L28 (-106.005, -102.0325) -> (-106.005, -133.02)
  spline S5 degree 3 poles (-111.7, -64.35) (-111.7, -65.5895) (-111.4137, -66.469) (-110.9068, -67.7094) (-110.1358, -69.5962) (-108.8783, -72.1868) (-107.8554, -77.2142) (-106.8228, -82.2895) (-106.005, -89.879) (-106.005, -102.0325) knots 0 0 0 0 0.246494 0.246494 0.246494 0.621459 0.621459 0.621459 1 1 1 1
  line L29 (-111.7, -64.35) -> (-111.7, -8.1693)
  line L30 (-1, -64.35) -> (-1, -8.1693)
  dimension "d229" = 2
  dimension "d235" = -1
  constraint coincident S1.end L11.start
  constraint coincident L2.end L8.start
  constraint coincident L2.start L6.start
  constraint parallel L8 L13
  constraint coincident L4.end L5.start
  constraint perpendicular L5 L14
  constraint coincident L18 L21.end
  constraint coincident L18 L22.end
  constraint coincident S0.end L23.start
  constraint coincident L25 L29.end
  constraint coincident L25 L30.end
extrude "Extrude36" add sketch "Sketch20" along normal up to near side of body 6 contours L0 L1 L2 L6 L8 L11 L12 L23 L24 S4 L26 L27 L28 S5 | L1 L6 S0 L19 L20 L25 S5 L29 | L1 L6 S5 | L1 S1 L8 L16 L17 L25 S4 L30 | L1 L8 S4 | L1 L6 S3 S5 | L1 L4 L5 S2 S3 L13 L14 L15 S4 L26 L27 L28 S5 | L6 S3 L22 L25 S5 L29 | L1 L8 S2 S4 | L8 S2 L21 L25 S4 L30 bodies 6
extrude "Extrude37" cut sketch "Sketch20" against normal blind 17.019 contours L0 L1 L6 S0 L10 L23 | L1 S0 L20 | L0 L1 S1 L8 L9 L11 L24 | L1 S1 L16 | L18 L19 L22 L25 | L17 L18 L21 L25 bodies 6
sketch "Sketch16" plane through (0, 0, 12.2) normal (0, 0, 1) x (-1, 0, 0)
  line L0 (-12.895, -129.09) -> (-99.805, -129.09)
  line L1 (-99.805, -129.09) -> (-99.805, -63.79)
  line L2 (-99.805, -63.79) -> (-12.895, -63.79)
  line L3 (-12.895, -63.79) -> (-12.895, -129.09)
  line L4 (-5.45, -6.29) -> (-5.45, -47.24)
  line L5 (-5.45, -47.24) -> (-107.25, -47.24)
  line L6 (-107.25, -47.24) -> (-107.25, -6.29)
  line L7 (-107.25, -6.29) -> (-5.45, -6.29)
  line L8 (-8.65, -49.36) -> (-8.65, -57.36)
  line L9 (-8.65, -57.36) -> (-107.25, -57.36)
  line L10 (-107.25, -57.36) -> (-107.25, -49.36)
  line L11 (-107.25, -49.36) -> (-8.65, -49.36)
  line L12 (-5.695, -134.02) -> (-5.695, -102.0325)
  spline S0 degree 3 poles (0, -64.35) (0, -65.4589) (-0.2155, -66.349) (-1.2269, -69.1321) (-2.3785, -71.1898) (-5.0573, -82.0909) (-5.695, -91.1433) (-5.695, -102.0325) knots 0 0 0 0 0.332673 0.332673 0.974518 0.974518 1.979375 1.979375 1.979375 1.979375
  line L13 (0, -64.35) -> (0, 0)
  line L14 (0, 0) -> (-112.7, 0)
  line L15 (-112.7, 0) -> (-112.7, -64.35)
  spline S1 degree 3 poles (-107.005, -102.0325) (-107.005, -87.4315) (-108.1871, -79.617) (-110.9745, -68.894) (-112.7, -67.4849) (-112.7, -64.35) knots 0 0 0 0 4.380314 4.380314 9.879234 9.879234 9.879234 9.879234
  line L16 (-107.005, -102.0325) -> (-107.005, -134.02)
  line L17 (-107.005, -134.02) -> (-5.695, -134.02)
  spline S2 degree 2 poles (-14.0855, -58.8018) (-13.8338, -58.8018) (-13.6094, -58.8802) knots 0 0 0 1 1 1
  spline S3 degree 2 poles (-13.6094, -58.8802) (-13.385, -58.9586) (-13.2153, -59.101) knots 0 0 0 1 1 1
  spline S4 degree 2 poles (-13.2153, -59.101) (-13.0455, -59.2435) (-12.96, -59.4382) knots 0 0 0 1 1 1
  line L18 (-12.96, -59.4382) -> (-13.5631, -59.6875)
  spline S5 degree 2 poles (-13.5631, -59.6875) (-13.632, -59.5854) (-13.7673, -59.4881) knots 0 0 0 1 1 1
  spline S6 degree 2 poles (-13.7673, -59.4881) (-13.9027, -59.3907) (-14.1116, -59.3907) knots 0 0 0 1 1 1
  spline S7 degree 2 poles (-14.1116, -59.3907) (-14.2066, -59.3907) (-14.2885, -59.4145) knots 0 0 0 1 1 1
  spline S8 degree 2 poles (-14.2885, -59.4145) (-14.3705, -59.4382) (-14.4203, -59.4833) knots 0 0 0 1 1 1
  spline S9 degree 2 poles (-14.4203, -59.4833) (-14.4702, -59.5284) (-14.4702, -59.5926) knots 0 0 0 1 1 1
  spline S10 degree 2 poles (-14.4702, -59.5926) (-14.4702, -59.678) (-14.3681, -59.7315) knots 0 0 0 1 1 1
  spline S11 degree 2 poles (-14.3681, -59.7315) (-14.266, -59.7849) (-14.1057, -59.8288) knots 0 0 0 1 1 1
  spline S12 degree 2 poles (-14.1057, -59.8288) (-13.9454, -59.8727) (-13.7638, -59.9274) knots 0 0 0 1 1 1
  spline S13 degree 2 poles (-13.7638, -59.9274) (-13.5821, -59.982) (-13.4218, -60.0686) knots 0 0 0 1 1 1
  spline S14 degree 2 poles (-13.4218, -60.0686) (-13.2616, -60.1553) (-13.1595, -60.2954) knots 0 0 0 1 1 1
  spline S15 degree 2 poles (-13.1595, -60.2954) (-13.0574, -60.4355) (-13.0574, -60.6516) knots 0 0 0 1 1 1
  spline S16 degree 2 poles (-13.0574, -60.6516) (-13.0574, -60.8914) (-13.1891, -61.0659) knots 0 0 0 1 1 1
  spline S17 degree 2 poles (-13.1891, -61.0659) (-13.3209, -61.2404) (-13.5501, -61.3366) knots 0 0 0 1 1 1
  spline S18 degree 2 poles (-13.5501, -61.3366) (-13.7792, -61.4328) (-14.0736, -61.4328) knots 0 0 0 1 1 1
  spline S19 degree 2 poles (-14.0736, -61.4328) (-14.4179, -61.4328) (-14.7017, -61.2844) knots 0 0 0 1 1 1
  spline S20 degree 2 poles (-14.7017, -61.2844) (-14.9854, -61.136) (-15.1089, -60.8772) knots 0 0 0 1 1 1
  line L19 (-15.1089, -60.8772) -> (-14.5106, -60.6278)
  spline S21 degree 2 poles (-14.5106, -60.6278) (-14.4464, -60.7204) (-14.336, -60.7845) knots 0 0 0 1 1 1
  spline S22 degree 2 poles (-14.336, -60.7845) (-14.2256, -60.8487) (-14.0641, -60.8487) knots 0 0 0 1 1 1
  spline S23 degree 2 poles (-14.0641, -60.8487) (-13.9264, -60.8487) (-13.8267, -60.7964) knots 0 0 0 1 1 1
  spline S24 degree 2 poles (-13.8267, -60.7964) (-13.727, -60.7442) (-13.727, -60.6492) knots 0 0 0 1 1 1
  spline S25 degree 2 poles (-13.727, -60.6492) (-13.727, -60.5613) (-13.8291, -60.5091) knots 0 0 0 1 1 1
  spline S26 degree 2 poles (-13.8291, -60.5091) (-13.9312, -60.4569) (-14.0926, -60.4165) knots 0 0 0 1 1 1
  spline S27 degree 2 poles (-14.0926, -60.4165) (-14.2541, -60.3761) (-14.4358, -60.3251) knots 0 0 0 1 1 1
  spline S28 degree 2 poles (-14.4358, -60.3251) (-14.6174, -60.274) (-14.7789, -60.1921) knots 0 0 0 1 1 1
  spline S29 degree 2 poles (-14.7789, -60.1921) (-14.9403, -60.1102) (-15.0424, -59.9748) knots 0 0 0 1 1 1
  spline S30 degree 2 poles (-15.0424, -59.9748) (-15.1445, -59.8395) (-15.1445, -59.6258) knots 0 0 0 1 1 1
  spline S31 degree 2 poles (-15.1445, -59.6258) (-15.1445, -59.3788) (-14.9997, -59.1925) knots 0 0 0 1 1 1
  spline S32 degree 2 poles (-14.9997, -59.1925) (-14.8549, -59.0061) (-14.615, -58.904) knots 0 0 0 1 1 1
  spline S33 degree 2 poles (-14.615, -58.904) (-14.3752, -58.8018) (-14.0855, -58.8018) knots 0 0 0 1 1 1
  spline S34 degree 2 poles (-17.0634, -58.8018) (-16.7072, -58.8018) (-16.4412, -58.9645) knots 0 0 0 1 1 1
  spline S35 degree 2 poles (-16.4412, -58.9645) (-16.1753, -59.1272) (-16.0305, -59.4228) knots 0 0 0 1 1 1
  spline S36 degree 2 poles (-16.0305, -59.4228) (-15.8856, -59.7184) (-15.8856, -60.1173) knots 0 0 0 1 1 1
  spline S37 degree 2 poles (-15.8856, -60.1173) (-15.8856, -60.5162) (-16.0305, -60.8119) knots 0 0 0 1 1 1
  spline S38 degree 2 poles (-16.0305, -60.8119) (-16.1753, -61.1075) (-16.4412, -61.2701) knots 0 0 0 1 1 1
  spline S39 degree 2 poles (-16.4412, -61.2701) (-16.7072, -61.4328) (-17.0634, -61.4328) knots 0 0 0 1 1 1
  spline S40 degree 2 poles (-17.0634, -61.4328) (-17.4195, -61.4328) (-17.6843, -61.2701) knots 0 0 0 1 1 1
  spline S41 degree 2 poles (-17.6843, -61.2701) (-17.9491, -61.1075) (-18.0951, -60.8119) knots 0 0 0 1 1 1
  spline S42 degree 2 poles (-18.0951, -60.8119) (-18.2411, -60.5162) (-18.2411, -60.1173) knots 0 0 0 1 1 1
  spline S43 degree 2 poles (-18.2411, -60.1173) (-18.2411, -59.7184) (-18.0951, -59.4228) knots 0 0 0 1 1 1
  spline S44 degree 2 poles (-18.0951, -59.4228) (-17.9491, -59.1272) (-17.6843, -58.9645) knots 0 0 0 1 1 1
  spline S45 degree 2 poles (-17.6843, -58.9645) (-17.4195, -58.8018) (-17.0634, -58.8018) knots 0 0 0 1 1 1
  spline S46 degree 2 poles (-17.0634, -59.443) (-17.2058, -59.443) (-17.3103, -59.5261) knots 0 0 0 1 1 1
  spline S47 degree 2 poles (-17.3103, -59.5261) (-17.4148, -59.6092) (-17.4718, -59.7611) knots 0 0 0 1 1 1
  spline S48 degree 2 poles (-17.4718, -59.7611) (-17.5288, -59.9131) (-17.5288, -60.1173) knots 0 0 0 1 1 1
  spline S49 degree 2 poles (-17.5288, -60.1173) (-17.5288, -60.3239) (-17.4718, -60.4747) knots 0 0 0 1 1 1
  spline S50 degree 2 poles (-17.4718, -60.4747) (-17.4148, -60.6255) (-17.3103, -60.7098) knots 0 0 0 1 1 1
  spline S51 degree 2 poles (-17.3103, -60.7098) (-17.2058, -60.794) (-17.0634, -60.794) knots 0 0 0 1 1 1
  spline S52 degree 2 poles (-17.0634, -60.794) (-16.9209, -60.794) (-16.8164, -60.7098) knots 0 0 0 1 1 1
  spline S53 degree 2 poles (-16.8164, -60.7098) (-16.7119, -60.6255) (-16.655, -60.4747) knots 0 0 0 1 1 1
  spline S54 degree 2 poles (-16.655, -60.4747) (-16.598, -60.3239) (-16.598, -60.1173) knots 0 0 0 1 1 1
  spline S55 degree 2 poles (-16.598, -60.1173) (-16.598, -59.9131) (-16.655, -59.7611) knots 0 0 0 1 1 1
  spline S56 degree 2 poles (-16.655, -59.7611) (-16.7119, -59.6092) (-16.8164, -59.5261) knots 0 0 0 1 1 1
  spline S57 degree 2 poles (-16.8164, -59.5261) (-16.9209, -59.443) (-17.0634, -59.443) knots 0 0 0 1 1 1
  spline S58 degree 2 poles (-20.3713, -58.8018) (-20.0578, -58.8018) (-19.8192, -58.9301) knots 0 0 0 1 1 1
  spline S59 degree 2 poles (-19.8192, -58.9301) (-19.5806, -59.0583) (-19.4452, -59.2851) knots 0 0 0 1 1 1
  spline S60 degree 2 poles (-19.4452, -59.2851) (-19.3099, -59.5118) (-19.3099, -59.811) knots 0 0 0 1 1 1
  line L20 (-19.3099, -59.811) -> (-19.3099, -62.4966)
  line L21 (-19.3099, -62.4966) -> (-20.0602, -62.4966)
  line L22 (-20.0602, -62.4966) -> (-20.0602, -59.8205)
  spline S61 degree 2 poles (-20.0602, -59.8205) (-20.0602, -59.6543) (-20.1789, -59.5498) knots 0 0 0 1 1 1
  spline S62 degree 2 poles (-20.1789, -59.5498) (-20.2977, -59.4453) (-20.4852, -59.4453) knots 0 0 0 1 1 1
  spline S63 degree 2 poles (-20.4852, -59.4453) (-20.604, -59.4453) (-20.7263, -59.4904) knots 0 0 0 1 1 1
  spline S64 degree 2 poles (-20.7263, -59.4904) (-20.8485, -59.5356) (-20.9435, -59.6163) knots 0 0 0 1 1 1
  line L23 (-20.9435, -59.6163) -> (-21.1976, -59.0132)
  spline S65 degree 2 poles (-21.1976, -59.0132) (-21.029, -58.9182) (-20.8046, -58.86) knots 0 0 0 1 1 1
  spline S66 degree 2 poles (-20.8046, -58.86) (-20.5802, -58.8018) (-20.3713, -58.8018) knots 0 0 0 1 1 1
  spline S67 degree 2 poles (-23.0832, -58.8018) (-22.8861, -58.8018) (-22.7519, -58.936) knots 0 0 0 1 1 1
  spline S68 degree 2 poles (-22.7519, -58.936) (-22.6178, -59.0702) (-22.6178, -59.2696) knots 0 0 0 1 1 1
  spline S69 degree 2 poles (-22.6178, -59.2696) (-22.6202, -59.4667) (-22.7531, -59.6009) knots 0 0 0 1 1 1
  spline S70 degree 2 poles (-22.7531, -59.6009) (-22.8861, -59.735) (-23.0808, -59.735) knots 0 0 0 1 1 1
  spline S71 degree 2 poles (-23.0808, -59.735) (-23.2803, -59.735) (-23.4156, -59.6009) knots 0 0 0 1 1 1
  spline S72 degree 2 poles (-23.4156, -59.6009) (-23.551, -59.4667) (-23.5533, -59.2696) knots 0 0 0 1 1 1
  spline S73 degree 2 poles (-23.5533, -59.2696) (-23.5533, -59.0702) (-23.4168, -58.936) knots 0 0 0 1 1 1
  spline S74 degree 2 poles (-23.4168, -58.936) (-23.2803, -58.8018) (-23.0832, -58.8018) knots 0 0 0 1 1 1
  spline S75 degree 2 poles (-26.4006, -58.8018) (-26.0278, -58.8018) (-25.769, -58.9823) knots 0 0 0 1 1 1
  spline S76 degree 2 poles (-25.769, -58.9823) (-25.5101, -59.1628) (-25.3748, -59.5142) knots 0 0 0 1 1 1
  spline S77 degree 2 poles (-25.3748, -59.5142) (-25.2395, -59.8656) (-25.2395, -60.3785) knots 0 0 0 1 1 1
  line L24 (-25.2395, -60.3785) -> (-25.2395, -60.7798)
  spline S78 degree 2 poles (-25.2395, -60.7798) (-25.2395, -61.2998) (-25.3748, -61.656) knots 0 0 0 1 1 1
  spline S79 degree 2 poles (-25.3748, -61.656) (-25.5101, -62.0122) (-25.769, -62.195) knots 0 0 0 1 1 1
  spline S80 degree 2 poles (-25.769, -62.195) (-26.0278, -62.3778) (-26.4006, -62.3778) knots 0 0 0 1 1 1
  spline S81 degree 2 poles (-26.4006, -62.3778) (-26.7734, -62.3778) (-27.0334, -62.195) knots 0 0 0 1 1 1
  spline S82 degree 2 poles (-27.0334, -62.195) (-27.2934, -62.0122) (-27.4275, -61.656) knots 0 0 0 1 1 1
  spline S83 degree 2 poles (-27.4275, -61.656) (-27.5617, -61.2998) (-27.5617, -60.7798) knots 0 0 0 1 1 1
  line L25 (-27.5617, -60.7798) -> (-27.5617, -60.3785)
  spline S84 degree 2 poles (-27.5617, -60.3785) (-27.5617, -59.8656) (-27.4275, -59.5142) knots 0 0 0 1 1 1
  spline S85 degree 2 poles (-27.4275, -59.5142) (-27.2934, -59.1628) (-27.0334, -58.9823) knots 0 0 0 1 1 1
  spline S86 degree 2 poles (-27.0334, -58.9823) (-26.7734, -58.8018) (-26.4006, -58.8018) knots 0 0 0 1 1 1
  spline S87 degree 2 poles (-26.4006, -59.4738) (-26.5407, -59.4738) (-26.6357, -59.5652) knots 0 0 0 1 1 1
  spline S88 degree 2 poles (-26.6357, -59.5652) (-26.7306, -59.6567) (-26.7793, -59.8324) knots 0 0 0 1 1 1
  spline S89 degree 2 poles (-26.7793, -59.8324) (-26.828, -60.0081) (-26.828, -60.2598) knots 0 0 0 1 1 1
  line L26 (-26.828, -60.2598) -> (-26.828, -60.9175)
  spline S90 degree 2 poles (-26.828, -60.9175) (-26.828, -61.1716) (-26.7793, -61.3473) knots 0 0 0 1 1 1
  spline S91 degree 2 poles (-26.7793, -61.3473) (-26.7306, -61.523) (-26.6357, -61.6144) knots 0 0 0 1 1 1
  spline S92 degree 2 poles (-26.6357, -61.6144) (-26.5407, -61.7059) (-26.4006, -61.7059) knots 0 0 0 1 1 1
  spline S93 degree 2 poles (-26.4006, -61.7059) (-26.2629, -61.7059) (-26.1679, -61.6156) knots 0 0 0 1 1 1
  spline S94 degree 2 poles (-26.1679, -61.6156) (-26.0729, -61.5254) (-26.023, -61.3497) knots 0 0 0 1 1 1
  spline S95 degree 2 poles (-26.023, -61.3497) (-25.9732, -61.174) (-25.9732, -60.9175) knots 0 0 0 1 1 1
  line L27 (-25.9732, -60.9175) -> (-25.9732, -60.2598)
  spline S96 degree 2 poles (-25.9732, -60.2598) (-25.9732, -60.0057) (-26.023, -59.83) knots 0 0 0 1 1 1
  spline S97 degree 2 poles (-26.023, -59.83) (-26.0729, -59.6543) (-26.1679, -59.5641) knots 0 0 0 1 1 1
  spline S98 degree 2 poles (-26.1679, -59.5641) (-26.2629, -59.4738) (-26.4006, -59.4738) knots 0 0 0 1 1 1
  line L28 (-25.7998, -59.7255) -> (-25.5101, -60.2004)
  line L29 (-25.5101, -60.2004) -> (-27.0132, -61.4447)
  line L30 (-27.0132, -61.4447) -> (-27.2886, -60.9816)
  line L31 (-27.2886, -60.9816) -> (-25.7998, -59.7255)
  line L32 (-29.1529, -58.8398) -> (-29.1529, -61.6417)
  line L33 (-29.1529, -61.6417) -> (-29.2929, -61.504)
  line L34 (-29.2929, -61.504) -> (-28.4548, -61.1455)
  line L35 (-28.4548, -61.1455) -> (-28.4548, -61.8721)
  line L36 (-28.4548, -61.8721) -> (-29.68, -62.3398)
  line L37 (-29.68, -62.3398) -> (-29.8889, -62.3398)
  line L38 (-29.8889, -62.3398) -> (-29.8889, -58.8398)
  line L39 (-29.8889, -58.8398) -> (-29.1529, -58.8398)
  line L40 (-28.4286, -58.8398) -> (-28.4286, -59.4904)
  line L41 (-28.4286, -59.4904) -> (-30.4754, -59.4904)
  line L42 (-30.4754, -59.4904) -> (-30.4754, -58.8398)
  line L43 (-30.4754, -58.8398) -> (-28.4286, -58.8398)